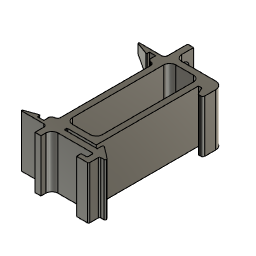
BuckConverterv3 (Autodesk Fusion 360 design; units mm, degrees)
Autodesk Fusion 360 part; units mm, degrees
other "Base Mesh Feature1" in component "buck din mount 5v"
sketch "Sketch1" plane through (0, 0, 0) normal (0, 0, 1) x (1, 0, 0) in component "buck din mount 5v"
  line L0 (14.8163, 45.1704) -> (26.2028, 45.1704)
  line L1 (28.7428, 42.6304) -> (28.7428, 38.9693)
  line L2 (28.1078, 38.3343) -> (27.5001, 38.3343)
  line L3 (26.9279, 38.694) -> (25.8969, 40.8368)
  line L4 (25.8969, 40.8368) -> (24.7705, 40.8368)
  line L5 (24.7705, 40.8368) -> (24.7705, 6.5829)
  line L6 (24.7705, 6.5829) -> (15.2022, 6.5829)
  line L7 (14.9722, 6.3529) -> (14.9722, 5.9121)
  line L8 (15.2022, 5.6821) -> (26.0152, 5.6821)
  line L9 (26.0152, 5.6821) -> (26.0152, 7.158)
  line L10 (26.6289, 7.4596) -> (30.5012, 4.4724)
  line L11 (30.6495, 4.1707) -> (30.6495, 4.077)
  line L12 (30.2685, 3.696) -> (29.1503, 3.696)
  line L13 (28.7693, 3.315) -> (28.7693, 0.396)
  line L14 (28.3883, 0.015) -> (24.7441, 0.015)
  line L15 (24.7441, 0.015) -> (24.7441, 1.5509)
  line L16 (24.7441, 1.5509) -> (26.3757, 1.5509)
  line L17 (26.7567, 1.9319) -> (26.7567, 3.2885)
  line L18 (26.3757, 3.6695) -> (14.8163, 3.6695)
  arc A0 (14.8163, 3.6695) -> (12.8163, 1.6695) centre (14.8163, 1.6695) ccw
  arc A1 (12.8163, 47.1704) -> (14.8163, 45.1704) centre (14.8163, 47.1704) ccw
  arc A2 (28.7428, 42.6304) -> (26.2028, 45.1704) centre (26.2028, 42.6304) ccw
  arc A3 (26.9279, 38.694) -> (27.5001, 38.3343) centre (27.5001, 38.9693) ccw
  arc A4 (28.1078, 38.3343) -> (28.7428, 38.9693) centre (28.1078, 38.9693) ccw
  arc A5 (26.6289, 7.4596) -> (26.0152, 7.158) centre (26.3962, 7.158) ccw
  arc A6 (30.6495, 4.1707) -> (30.5012, 4.4724) centre (30.2685, 4.1707) ccw
  arc A7 (30.2685, 3.696) -> (30.6495, 4.077) centre (30.2685, 4.077) ccw
  arc A8 (29.1503, 3.696) -> (28.7693, 3.315) centre (29.1503, 3.315) ccw
  arc A9 (28.3883, 0.015) -> (28.7693, 0.396) centre (28.3883, 0.396) ccw
  arc A10 (26.3757, 1.5509) -> (26.7567, 1.9319) centre (26.3757, 1.9319) ccw
  arc A11 (26.7567, 3.2885) -> (26.3757, 3.6695) centre (26.3757, 3.2885) ccw
  line L19 (2.2872, 43.0719) -> (6.4479, 41.5576)
  line L20 (6.7163, 41.7455) -> (6.7163, 42.4599)
  line L21 (6.7163, 42.4599) -> (8.8163, 42.4599)
  line L22 (8.8163, 42.4599) -> (8.8163, 40.5599)
  line L23 (12.8163, 47.1704) -> (12.8163, 51.1704)
  line L24 (12.8163, 51.1704) -> (10.8163, 51.1704)
  line L25 (10.8163, 51.1704) -> (10.8163, 44.4599)
  line L26 (9.8163, 43.4599) -> (2.3556, 43.4599)
  line L27 (10.8163, 0.015) -> (12.8163, 0.015)
  line L28 (12.8163, 0.015) -> (12.8163, 1.6695)
  line L29 (24.7705, 23.7099) -> (-6.7901, 23.7099) construction
  arc A12 (9.8163, 43.4599) -> (10.8163, 44.4599) centre (9.8163, 44.4599) ccw
  arc A13 (6.4479, 41.5576) -> (6.7163, 41.7455) centre (6.5163, 41.7455) ccw
  arc A14 (2.3556, 43.4599) -> (2.2872, 43.0719) centre (2.3556, 43.2599) ccw
  line L30 (10.8163, 0.015) -> (10.8163, 2.9599)
  line L31 (10.8163, 8.5599) -> (10.8163, 38.8599)
  line L32 (9.5163, 39.8599) -> (9.8163, 39.8599)
  arc A15 (10.8163, 38.8599) -> (9.8163, 39.8599) centre (9.8163, 38.8599) ccw
  line L33 (9.5163, 39.8599) -> (8.8163, 40.5599)
  line L34 (6.7163, 5.6742) -> (6.7163, 4.9599)
  arc A16 (9.8163, 7.5599) -> (10.8163, 8.5599) centre (9.8163, 8.5599) ccw
  line L35 (9.5163, 7.5599) -> (9.8163, 7.5599)
  arc A17 (6.7163, 5.6742) -> (6.4479, 5.8622) centre (6.5163, 5.6742) ccw
  line L36 (9.5163, 7.5599) -> (8.8163, 6.8599)
  arc A18 (10.8163, 2.9599) -> (9.8163, 3.9599) centre (9.8163, 2.9599) ccw
  line L37 (6.7163, 4.9599) -> (8.8163, 4.9599)
  line L38 (2.2872, 4.3478) -> (6.4479, 5.8622)
  line L39 (9.8163, 3.9599) -> (2.3556, 3.9599)
  arc A19 (2.2872, 4.3478) -> (2.3556, 3.9599) centre (2.3556, 4.1599) ccw
  line L40 (8.8163, 4.9599) -> (8.8163, 6.8599)
  line L41 (14.8163, 43.1704) -> (20.7705, 43.1704)
  line L42 (22.7705, 41.1704) -> (22.7705, 10.5829)
  line L43 (20.7705, 8.5829) -> (14.8163, 8.5829)
  line L44 (12.8163, 10.5829) -> (12.8163, 41.1704)
  arc A20 (14.8163, 43.1704) -> (12.8163, 41.1704) centre (14.8163, 41.1704) ccw
  arc A21 (22.7705, 41.1704) -> (20.7705, 43.1704) centre (20.7705, 41.1704) ccw
  arc A22 (20.7705, 8.5829) -> (22.7705, 10.5829) centre (20.7705, 10.5829) ccw
  arc A23 (12.8163, 10.5829) -> (14.8163, 8.5829) centre (14.8163, 10.5829) ccw
  arc A24 (15.2022, 6.5829) -> (14.9722, 6.3529) centre (15.2022, 6.3529) ccw
  arc A25 (14.9722, 5.9121) -> (15.2022, 5.6821) centre (15.2022, 5.9121) ccw
  point P0 (6.7163, 41.4599)
  point P1 (8.8163, 39.3264)
  point P2 (8.8163, 39.8599)
  point P3 (8.8163, 7.5599)
  point P4 (6.7163, 5.9599)
  point P5 (8.8163, 8.0933)
  dimension "d1" = 2
  dimension "d2" = 2.54
  dimension "d3" = 0.635
  dimension "d4" = 0.381
  dimension "d78" = 2
  dimension "d82" = 18.75
  dimension "d83" = 4.3336
  dimension "d84" = 0.9008
  dimension "d86" = 0.2
  dimension "d87" = 0.2
  dimension "d90" = 1
  dimension "d91" = 2
  dimension "d92" = 2.1
  dimension "d93" = 1
  dimension "d94" = 2.6
  dimension "d95" = 20
  dimension "d96" = 6
  dimension "d97" = 1
  dimension "d98" = 0.7
  dimension "d99" = 0.7
  dimension "d100" = 2
  dimension "d101" = 2
  dimension "d102" = 2
  dimension "d103" = 2
  dimension "d106" = 0.23
  dimension "d117" = 2
  constraint vertical L30
  constraint perpendicular L0 L1
  constraint perpendicular L1 L2
  constraint perpendicular L1 L4
  constraint perpendicular L4 L5
  constraint perpendicular L5 L6
  constraint perpendicular L6 L7
  constraint perpendicular L5 L8
  constraint perpendicular L8 L9
  constraint perpendicular L8 L11
  constraint perpendicular L11 L12
  constraint perpendicular L12 L13
  constraint perpendicular L13 L14
  constraint perpendicular L14 L15
  constraint perpendicular L15 L16
  constraint perpendicular L16 L17
  constraint tangent L18 A0
  constraint tangent L0 A1
  constraint equal A0 A1
  constraint tangent L0 A2
  constraint tangent L1 A2
  constraint tangent L2 A3
  constraint tangent L3 A3
  constraint tangent L1 A4
  constraint tangent L2 A4
  constraint equal A3 A4
  constraint tangent L9 A5
  constraint tangent L10 A5
  constraint tangent L10 A6
  constraint tangent L11 A6
  constraint equal A5 A6
  constraint tangent L11 A7
  constraint tangent L12 A7
  constraint equal A5 A7
  constraint tangent L13 A8
  constraint tangent L12 A8
  constraint equal A5 A8
  constraint tangent L13 A9
  constraint tangent L14 A9
  constraint equal A5 A9
  constraint tangent L16 A10
  constraint tangent L17 A10
  constraint equal A5 A10
  constraint tangent L17 A11
  constraint tangent L18 A11
  constraint equal A5 A11
  constraint perpendicular L20 L21
  constraint perpendicular L21 L22
  constraint tangent A1 L23
  constraint vertical L23
  constraint perpendicular L23 L24
  constraint perpendicular L24 L25
  constraint horizontal L26
  constraint vertical L28
  constraint midpoint L5 L29.start
  constraint perpendicular L29 L30
  constraint tangent L26 A12
  constraint tangent L25 A12
  constraint coincident P0 L20
  constraint coincident P0 L19
  constraint tangent L20 A13
  constraint tangent L19 A13
  constraint tangent L19 A14
  constraint tangent L26 A14
  constraint coincident P1 L22
  constraint symmetric L29 L25.end L30.end
  constraint collinear L30 L31
  constraint tangent A0 L28
  constraint collinear L14 L27
  constraint tangent L31 A15
  constraint tangent L32 A15
  constraint equal A12 A15
  constraint horizontal L32
  constraint coincident P2 L32
  constraint coincident L22 P2
  constraint symmetric P0 L29 P4
  constraint symmetric L20.end L29 L34.end
  constraint symmetric L21.end L29 L37.end
  constraint symmetric P1 L29 P5
  constraint symmetric L29 L26.start A18.end
  constraint symmetric L29 A12 A18
  constraint symmetric L29 L20.start L34.start
  constraint symmetric L29 L19.end A17.end
  constraint symmetric L29 A13 A17
  constraint symmetric L29 L19.start L38.start
  constraint symmetric L29 L26.end L39.end
  constraint symmetric L29 A14 A19
  constraint symmetric L29 P2 P3
  constraint symmetric L29 L31.end L31.start
  constraint symmetric L29 L32.end A16.start
  constraint symmetric L29 A15 A16
  constraint symmetric L29 L32.start L35.start
  constraint symmetric L29 L22.end L36.end
  constraint horizontal L41
  constraint vertical L42
  constraint horizontal L43
  constraint vertical L44
  constraint collinear L23 L44
  constraint tangent L44 A20
  constraint tangent L41 A20
  constraint tangent L41 A21
  constraint tangent L42 A21
  constraint equal A20 A21
  constraint tangent L42 A22
  constraint tangent L43 A22
  constraint equal A20 A22
  constraint tangent L43 A23
  constraint tangent L44 A23
  constraint equal A20 A23
  constraint tangent L6 A24
  constraint tangent L7 A24
  constraint tangent L7 A25
  constraint tangent L8 A25
  constraint equal A24 A25
  measures "d1" radius of A0
  measures "d2" radius of A2
  measures "d3" radius of A3
  measures "d4" radius of A5
  measures "d78" distance of L23.end L24.end
  measures "d82" distance of L21 L29
  measures "d83" distance of L0 L4
  measures "d84" distance of L6 L8
  measures "d86" radius of A13
  measures "d87" radius of A14
  measures "d90" distance of L21 L26
  measures "d91" distance of L22 L31
  measures "d92" distance of L20.end L21.end
  measures "d93" distance of P0 L21
  measures "d94" distance of L21.end P2
  measures "d95" angle of L19 L26
  measures "d96" distance of L0 L24
  measures "d97" radius of A15
  measures "d98" distance of P2 L32.start
  measures "d99" distance of P2 L22.end
  measures "d100" distance of L0 L41
  measures "d101" distance of L5 L42
  measures "d102" distance of L6 L43
  measures "d103" radius of A20
  measures "d106" radius of A24
  measures "d117" distance of L27.start L27.end
extrude "Extrude3" add sketch "Sketch1" along normal blind 17.5
sketch "Sketch8" plane through (10.8163, 0, 0) normal (-1, 0, 0) x (0, -1, 0)
  line L0 (-51.1704, 0) -> (-44.4599, 0)
  line L1 (-44.4599, 0) -> (-44.4599, 17.5)
  line L2 (-44.4599, 17.5) -> (-51.1704, 17.5)
  line L3 (-51.1704, 17.5) -> (-51.1704, 0)
  line L4 (-47.8151, 17.5) -> (-47.8151, 0) construction
  circle A0 centre (-47.8151, 13.05) radius 1.8
  circle A1 centre (-47.8151, 4.45) radius 1.8
  line L5 (-44.4599, 8.75) -> (-51.1704, 8.75) construction
  point P0 (-47.8151, 11.25)
  dimension "d107" = 3.6
  dimension "d109" = 2.5
  constraint midpoint L2 L4.start
  constraint midpoint L0 L4.end
  constraint coincident L4 A0.centre
  constraint coincident L4 A1.centre
  constraint equal A0 A1
  constraint midpoint L1 L5.start
  constraint midpoint L3 L5.end
  constraint symmetric A0.centre A1.centre L5
  constraint coincident A0 P0
  constraint coincident L4 P0
  measures "d107" diameter of A0
  measures "d109" distance of L5 P0
extrude "Extrude4" cut sketch "Sketch8" against normal blind 6 contours A0 | A1
sketch "Sketch9" plane through (0, 43.4599, 0) normal (0, 1, 0) x (-1, 0, 0)
  line L0 (-9.8163, 0) -> (-2.3556, 0)
  line L1 (-2.3556, 0) -> (-2.3556, 17.5)
  line L2 (-2.3556, 17.5) -> (-9.8163, 17.5)
  line L3 (-9.8163, 17.5) -> (-9.8163, 0)
  line L4 (-6.4479, 0) -> (-6.4479, 17.5)
  line L5 (-1.4479, 2.3936) -> (-5.4479, 5.75)
  line L6 (-5.4479, 5.75) -> (-5.4479, 11.75)
  line L7 (-5.4479, 11.75) -> (-1.4479, 15.1064)
  line L8 (-1.4479, 15.1064) -> (-1.4479, 2.3936)
  line L9 (-6.4479, 8.75) -> (1.1683, 8.75) construction
  point P0 (-5.4479, 8.75)
  dimension "d112" = 130
  dimension "d113" = 130
  dimension "d114" = 1
  dimension "d115" = 4
  dimension "d116" = 6
  constraint parallel L1 L6
  constraint vertical L8
  constraint midpoint L4 L9.start
  constraint perpendicular L8 L9
  constraint midpoint L6 P0
  constraint coincident L9 P0
  measures "d112" angle of L5 L6
  measures "d113" angle of L6 L7
  measures "d114" distance of L4 L6
  measures "d115" distance of L6 L8
  measures "d116" distance of L5.end L6.end
extrude "Extrude5" cut sketch "Sketch9" against normal blind 4 contours L1 L5 L6 L7 | L1 L5 L7 L8
component "buck din mount 5v" placed x (1, 0, 0) y (0, 1, 0) z (0, 0, 1) at (0, 0, 0)
equation "d82 = ( 37.5 / 2 ) * 1 mm"
equation "d99 = d98"
